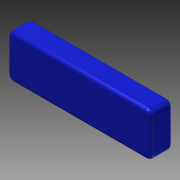
# Autodesk Inventor part: Batteri
Saved by Autodesk Inventor 2015 (Build 190159000, 159)
## iProperties
Created: 2015-06-20
Part Number: Batteri
Material: Aluminum 6061
Document SubType Name: Modeling
Designer: Kristian
Mass: 294.193 g
Surface Area: 170.03 cm^2
Volume: 108.961 cm^3
Density: 2.7 g/cm^3
Appearance: Blue - Wall Paint - Glossy
Author: Kristian
Autodesk Inventor part; units mm, degrees
ref_plane "YZ Plane" through (0, 0, 0) normal (1, 0, 0) x (0, 1, 0)
ref_plane "XZ Plane" through (0, 0, 0) normal (0, 1, 0) x (-1, 0, 0)
ref_plane "XY Plane" through (0, 0, 0) normal (0, 0, 1) x (1, 0, 0)
sketch "Sketch1" plane through (0, 0, 0) normal (0, 1, 0) x (-1, 0, 0)
  line L0 (-67.5, 20.5) -> (67.5, 20.5)
  line L1 (67.5, 20.5) -> (67.5, -20.5)
  line L2 (67.5, -20.5) -> (-67.5, -20.5)
  line L3 (-67.5, -20.5) -> (-67.5, 20.5)
  line L4 (-67.5, 20.5) -> (67.5, -20.5) construction
  line L5 (67.5, 20.5) -> (-67.5, -20.5) construction
  point P0 (0, 0)
  dimension "d0" = 135
  dimension "d1" = 41
  constraints: 12 end point, 2 midpoint, 2 parallel, 1 horizontal, 1 perpendicular
  measures "d0" distance of L1.end L2.end
  measures "d1" distance of L0.end L1.end
extrude "Extrusion1" add sketch "Sketch1" along normal blind 20
fillet "Fillet1" radius 5 4 edges at (-67.5, 10, 20.5) (-67.5, 10, -20.5) (67.5, 10, -20.5) (67.5, 10, 20.5)
fillet "Fillet2" radius 3 16 edges at (66.0355, 20, 19.0355) (67.5, 20, 0) (66.0355, 20, -19.0355) (0, 20, -20.5) (-66.0355, 20, -19.0355) (-67.5, 20, 0) (-66.0355, 20, 19.0355) (0, 20, 20.5) (-66.0355, 0, 19.0355) (-67.5, 0, 0) (-66.0355, 0, -19.0355) (0, 0, -20.5) (66.0355, 0, -19.0355) (67.5, 0, 0) (66.0355, 0, 19.0355) (0, 0, 20.5)
body "Solid1"
